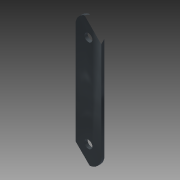
# Autodesk Inventor part: KreplenieBoltam
Saved by Autodesk Inventor 2015 (Build 190159000, 159)
## iProperties
Created: 2016-05-21
Part Number: KreplenieBoltam
Material: Iron, Cast
Document SubType Name: Modeling
Designer: Kostya
Density: 7.15 g/cm^3
Appearance: Iron Gray
Author: Kostya
Autodesk Inventor part; units mm, degrees
ref_plane "YZ Plane" through (0, 0, 0) normal (1, 0, 0) x (0, 1, 0)
ref_plane "XZ Plane" through (0, 0, 0) normal (0, 1, 0) x (-1, 0, 0)
ref_plane "XY Plane" through (0, 0, 0) normal (0, 0, 1) x (1, 0, 0)
sketch "Sketch1" plane through (0, 0, 0) normal (0, 1, 0) x (-1, 0, 0)
  circle A0 centre (0, -18) radius 1.55
  circle A1 centre (0, 18) radius 1.55
  line L0 (0, 25) -> (0, 25)
  line L1 (-5, 20) -> (-5, -20)
  line L2 (0, -25) -> (0, -25)
  line L3 (5, -20) -> (5, 20)
  arc A2 (5, 20) -> (0, 25) centre (0, 20) ccw
  arc A3 (0, 25) -> (-5, 20) centre (0, 20) ccw
  arc A4 (-5, -20) -> (0, -25) centre (0, -20) ccw
  arc A5 (0, -25) -> (5, -20) centre (0, -20) ccw
  point P0 (0, 0)
  point P1 (-5, -25)
  point P2 (-5, 25)
  point P3 (5, -25)
  point P4 (0, -25)
  dimension "d0" = 3.1
  dimension "d1" = 3.1
  dimension "d2" = 10
  dimension "d3" = 50
  dimension "d4" = 5
  constraints: 8 end point, 8 point on circle, 8 tangent, 6 centre point, 6 point on line, 3 equal radius, 2 parallel, 1 horizontal, 1 midpoint, 1 perpendicular, 1 vertical alignment
  measures "d0" diameter of A0
  measures "d1" diameter of A1
  measures "d2" distance of point (5, -25) point (-5, -25)
  measures "d3" distance of point (-5, -25) point (-5, 25)
  measures "d4" radius of A2
extrude "Extrusion1" add sketch "Sketch1" along normal blind 1.25
body "Solid1"
